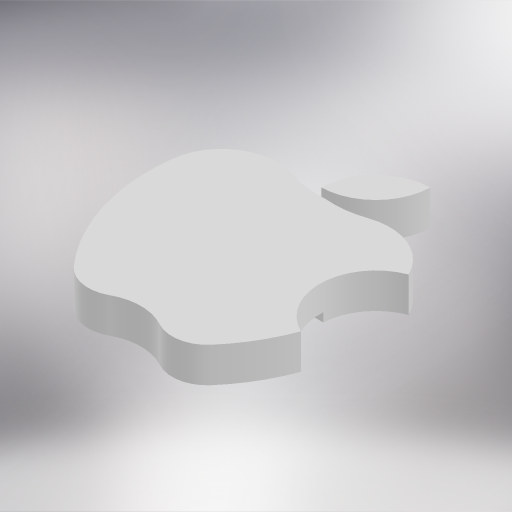
# Autodesk Inventor part: Apple_logo_white
Saved by Autodesk Inventor 2024 (Build 280153000, 153)
## iProperties
Created: 2023-10-30
Part Number: Apple_logo_white
Material: Generic
Document SubType Name: Modeling
Designer: SSAFY
Density: 1 g/cm^3
Appearance: Default
Author: SSAFY
Autodesk Inventor part; units mm, degrees
ref_plane "YZ Plane" through (0, 0, 0) normal (1, 0, 0) x (0, 1, 0)
ref_plane "XZ Plane" through (0, 0, 0) normal (0, 1, 0) x (-1, 0, 0)
ref_plane "XY Plane" through (0, 0, 0) normal (0, 0, 1) x (1, 0, 0)
sketch "Sketch2" plane through (0, 0, 0) normal (0, 1, 0) x (-1, 0, 0)
  line L0 (0, 0) -> (-15.380673, 0) construction
  line L1 (0, 12) -> (0, -86.646063) construction
  circle A0 centre (0, 0) radius 2
  circle A1 centre (-12, 0) radius 10
  circle A2 centre (-23.313708, -11.313708) radius 6
  circle A3 centre (-16, -32.062435) radius 16
  line L2 (-16, -48.062435) -> (0, -48.062435)
  line L3 (-12, 10) -> (0, 10)
  line L4 (-12, 0) -> (-23.313708, -11.313708)
  arc A4 (-19.562803, 6.542477) -> (-31.877188, -34.041046) centre (19.892258, -27.589553) ccw
  line L5 (0, 0) -> (15.380673, 0) construction
  circle A5 centre (0, 0) radius 2
  circle A6 centre (12, 0) radius 10
  circle A7 centre (23.313708, -11.313708) radius 6
  circle A8 centre (16, -32.062435) radius 16
  line L6 (16, -48.062435) -> (0, -48.062435)
  line L7 (12, 10) -> (0, 10)
  line L8 (12, 0) -> (23.313708, -11.313708)
  arc A9 (31.877188, -34.041046) -> (19.562803, 6.542477) centre (-19.892258, -27.589553) ccw
  arc A10 (10.751933, -47.177256) -> (0, -45.834116) centre (2.223823, -71.738838) ccw
  arc A11 (0, 6.931712) -> (7.2, 8.772685) centre (0, 21.931712) ccw
  arc A12 (0, -45.834116) -> (-10.751933, -47.177256) centre (-2.223823, -71.738838) ccw
  arc A13 (-7.2, 8.772685) -> (0, 6.931712) centre (0, 21.931712) ccw
  line L9 (-23.313708, -11.313708) -> (-58.366086, -46.366086)
  line L10 (-12, 0) -> (-38.351414, 26.351414)
  line L11 (10.154637, -70.237898) -> (-38.67512, -21.408141)
  circle A14 centre (-36.041631, -24.041631) radius 16
  circle A15 centre (-12.425271, -47.65799) radius 16
  circle A16 centre (3.979174, -64.062435) radius 16
  point P0 (3.569483, -48.067681)
  point P1 (-12.01558, -63.652744)
  point P2 (-7.2, 8.772685)
  point P3 (-29.089266, -9.631057)
  point P4 (-30.409272, -39.017496)
  point P5 (-10.751933, -47.177256)
  dimension "d0" = 4
  dimension "d1" = 20
  dimension "d2" = 12
  dimension "d3" = 32
  dimension "d4" = 135
  dimension "d6" = 26
  dimension "d7" = 15
  dimension "d8" = 90
  dimension "d12" = 34
  dimension "d13" = 32
  dimension "d14" = 32
  dimension "d15" = 32
  constraints: 24 end point, 24 point on circle, 17 centre point, 13 symmetric about line, 13 tangent, 11 point on line, 2 coincident, 2 horizontal, 1 collinear, 1 parallel, 1 vertical, 7 other
  measures "d0" diameter of A0
  measures "d1" diameter of A1
  measures "d2" diameter of A2
  measures "d3" diameter of A3
  measures "d4" angle of L4 L0
  measures "d6" radius of A10
  measures "d7" radius of A11
  measures "d8" angle of L10 L4
  measures "d12" distance between parallel lines of L10 L11
  measures "d13" diameter of A14
  measures "d14" diameter of A15
  measures "d15" diameter of A16
sketch "Sketch2 outline for Extrusion1" plane through (0, 0, 0) normal (0, 1, 0) x (-1, 0, 0)
  arc A0 (3.569483, -48.067681) -> (-12.01558, -63.652744) centre (3.979174, -64.062435) ccw
  arc A1 (-12.01558, -63.652744) -> (3.569483, -48.067681) centre (-12.425271, -47.65799) ccw
  arc A2 (31.877188, -34.041046) -> (19.562803, 6.542477) centre (-19.892258, -27.589553) ccw
  arc A3 (19.562803, 6.542477) -> (7.2, 8.772685) centre (12, 0) ccw
  arc A4 (7.2, 8.772685) -> (-7.2, 8.772685) centre (0, 21.931712) cw
  arc A5 (-7.2, 8.772685) -> (-19.562803, 6.542477) centre (-12, 0) ccw
  arc A6 (-19.562803, 6.542477) -> (-29.089266, -9.631057) centre (19.892258, -27.589553) ccw
  arc A7 (-29.089266, -9.631057) -> (-30.409272, -39.017496) centre (-36.041631, -24.041631) cw
  arc A8 (-30.409272, -39.017496) -> (-10.751933, -47.177256) centre (-16, -32.062435) ccw
  arc A9 (-10.751933, -47.177256) -> (0, -45.834116) centre (-2.223823, -71.738838) cw
  arc A10 (0, -45.834116) -> (10.751933, -47.177256) centre (2.223823, -71.738838) cw
  arc A11 (10.751933, -47.177256) -> (31.877188, -34.041046) centre (16, -32.062435) ccw
extrude "Extrusion1" add sketch "Sketch2 outline for Extrusion1" along normal blind 10
sketch "Sketch3" plane through (0, 0, 0) normal (0, -1, 0) x (1, 0, 0)
  line L0 (-51.381118, -10) -> (56.260395, -10)
  line L1 (56.260395, -10) -> (56.260395, -25)
  line L2 (56.260395, -25) -> (-51.381118, -25)
  line L3 (-51.381118, -25) -> (-51.381118, -10)
  point P0 (0, 0)
  dimension "d22" = 15
  dimension "d23" = 10
  constraints: 8 end point, 2 parallel, 1 horizontal, 1 perpendicular
  measures "d22" distance of L0.end L1.end
  measures "d23" distance from line of L0 point (0, 0)
extrude "Extrusion2" cut sketch "Sketch3" against normal blind 2.5
body "Solid1"
